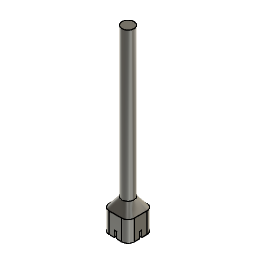
cube-connector-shaft (Autodesk Fusion 360 design; units mm, degrees)
Autodesk Fusion 360 part; units mm, degrees
sketch "Sketch1" plane through (0, 0, 0) normal (0, 0, 1) x (1, 0, 0) in component "Cube Connector"
  line L0 (4, 0) -> (12, 0)
  line L1 (16, 4) -> (16, 12)
  line L2 (12, 16) -> (4, 16)
  line L3 (0, 12) -> (0, 4)
  arc A0 (12, 0) -> (16, 4) centre (12, 4) ccw
  arc A1 (0, 4) -> (4, 0) centre (4, 4) ccw
  arc A2 (4, 16) -> (0, 12) centre (4, 12) ccw
  arc A3 (16, 12) -> (12, 16) centre (12, 12) ccw
  circle A4 centre (8, 8) radius 5.375
  point P0 (16, 0)
  point P1 (0, 16)
  dimension "d83" = 16
  dimension "d84" = 16
  dimension "d85" = 4
  dimension "d86" = 10.75
  constraint horizontal L0
  constraint vertical L1
  constraint horizontal L2
  constraint vertical L3
  constraint coincident P0 L0
  constraint coincident P0 L1
  constraint tangent L0 A0
  constraint tangent L1 A0
  constraint coincident origin L0
  constraint coincident origin L3
  constraint tangent L0 A1
  constraint tangent L3 A1
  constraint equal A0 A1
  constraint coincident P1 L2
  constraint coincident P1 L3
  constraint tangent L2 A2
  constraint tangent L3 A2
  constraint equal A0 A2
  constraint tangent L1 A3
  constraint tangent L2 A3
  constraint equal A0 A3
  measures "d83" distance of origin P0
  measures "d84" distance of origin P1
  measures "d85" radius of A0
  measures "d86" diameter of A4
extrude "Extrude1" add sketch "Sketch1" along normal blind 13 contours L0 L1 L2 L3 A0 A1 A2 A3 | A4 makes body 1 in component "Cube Connector"
extrude "Extrude2" cut sketch "Sketch1" along normal blind 11 contours A4 bodies 1 in component "Cube Connector"
sketch "Sketch6" plane through (0, 0, 13) normal (0, 0, 1) x (-1, 0, 0) in component "Cube Connector"
  arc A0 (-16, -12) -> (-12, -16) centre (-12, -12) ccw
  line L0 (-12, -16) -> (-4, -16)
  arc A1 (-4, -16) -> (0, -12) centre (-4, -12) ccw
  line L1 (0, -12) -> (0, -4)
  arc A2 (0, -4) -> (-4, 0) centre (-4, -4) ccw
  line L2 (-4, 0) -> (-12, 0)
  arc A3 (-12, 0) -> (-16, -4) centre (-12, -4) ccw
  line L3 (-16, -4) -> (-16, -12)
  circle A4 centre (-8, -8) radius 3.875
  dimension "d98" = 7.75
  measures "d98" diameter of A4
extrude "Extrude5" add sketch "Sketch6" along normal blind 100 separate body contours A4 makes body 2 in component "Cube Connector"
ref_plane "WorkPlane2" through (8, 8, 19) normal (0, 0, 1) x (-1, 0, 0) in component "Cube Connector"
sketch "Sketch27" plane through (8, 8, 19) normal (0, 0, 1) x (1, 0, 0)
  circle A0 centre (0, 0) radius 3.875
  dimension "d115" = 7.75
  constraint coincident A0.centre origin
  measures "d115" diameter of A0
sketch "Sketch14" plane through (8, 8, 19) normal (0, 0, 1) x (1, 0, 0) in component "Cube Connector"
  circle A0 centre (0, 0) radius 3.875
  dimension "d116" = 7.75
  constraint coincident A0.centre origin
  measures "d116" diameter of A0
loft "Loft2" add profiles "Sketch6", "Sketch14" section 1 section 2 separate body makes body 3 in component "Cube Connector"
sketch "Sketch16" plane through (0, 0, 0) normal (0, 0, 1) x (1, 0, 0) in component "Cube Connector"
  line L0 (16, 8.75) -> (0, 8.75)
  arc A0 (0, 8.75) -> (0, 7.25) centre (0, 8) ccw
  line L1 (0, 7.25) -> (16, 7.25)
  arc A1 (16, 7.25) -> (16, 8.75) centre (16, 8) ccw
  line L2 (16, 8) -> (0, 8) construction
  line L3 (7.25, 16) -> (7.25, 0)
  arc A2 (7.25, 0) -> (8.75, 0) centre (8, 0) ccw
  line L4 (8.75, 0) -> (8.75, 16)
  arc A3 (8.75, 16) -> (7.25, 16) centre (8, 16) ccw
  line L5 (8, 16) -> (8, 0) construction
  dimension "d120" = 1.5
  dimension "d121" = 1.5
  constraint tangent L0 A0
  constraint tangent A0 L1
  constraint parallel L0 L1
  constraint tangent L1 A1
  constraint tangent L0 A1
  constraint horizontal L2
  constraint tangent L3 A2
  constraint tangent A2 L4
  constraint parallel L3 L4
  constraint tangent L4 A3
  constraint tangent L3 A3
  constraint vertical L5
  measures "d120" diameter of A0
  measures "d121" diameter of A2
extrude "Extrude6" cut sketch "Sketch16" along normal blind 4 bodies 1 in component "Cube Connector"
sketch "Sketch14 (2)" plane through (0, 0, 0) normal (0, 0, 1) x (1, 0, 0)
  circle A0 through (0.75, 7.75, 43) (11.25, 1.6878, 43) (11.25, 13.8122, 43)
  circle A1 through (4.25, 7.75, 43) (9.5, 4.7189, 43) (9.5, 10.7811, 43)
  line L0 (7.4024, 0.7586, 43) -> (7.4024, 4.2673, 43)
  line L1 (7.4024, 4.2673, 43) -> (7.4024, 4.2805, 37)
  line L2 (7.4024, 0.7586, 43) -> (7.4024, 4.2805, 37)
  dimension "d53" = 6
revolve "Revolve3" [suppressed]
delete_face "DeleteFace3" [suppressed]
sketch "Sketch17" plane through (0, 0, 43) normal (0, 0, -1) x (1, 0, 0)
  circle A0 centre (7.75, -7.75) radius 7
  circle A1 centre (7.75, -7.75) radius 3.5
  circle A2 through (13.25, -7.75, 32) (5, -2.9869, 32) (5, -12.5131, 32)
  line L0 (7.75, -7.75, 0) -> (7.75, -7.75, 32)
  line L1 (6.8215, -14.6882) -> (7.4028, -11.2327)
  line L2 (7.4028, -11.2327, 0) -> (7.4028, -11.2327, 24.04)
  line L3 (6.8215, -14.6882, 0) -> (7.4028, -11.2327, 5.0784)
  point P0 (6.8215, -14.6882)
  point P1 (7.4028, -11.2327)
  dimension "d57" = 24.04
  constraint coincident A0.centre A1.centre
  constraint coincident P0 L1.start
  constraint coincident P1 L1.end
  measures "d57" distance of P1 L1.end
component "Cube Connector" placed x (1, 0, 0) y (0, 1, 0) z (0, 0, 1) at (0, 0, 0)
named bodies: "Base", "Shaft", "Loft"
